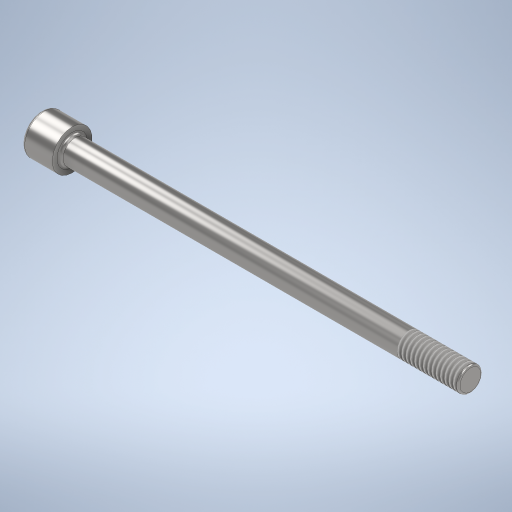
# Autodesk Inventor part: m4x70_example
Saved by Autodesk Inventor 2024 (Build 280153000, 153)
## iProperties
Created: 2025-12-19
Part Number: m4x70_example
Material: Stainless Steel
Document SubType Name: Modeling
Designer: schar
Density: 8 g/cm^3
Appearance: Semi-Polished
Author: schar
Autodesk Inventor part; units mm, degrees
ref_plane "YZ Plane" through (0, 0, 0) normal (1, 0, 0) x (0, 1, 0)
ref_plane "XZ Plane" through (0, 0, 0) normal (0, 1, 0) x (-1, 0, 0)
ref_plane "XY Plane" through (0, 0, 0) normal (0, 0, 1) x (1, 0, 0)
sketch "Sketch1" plane through (0, 0, 0) normal (1, 0, 0) x (0, 1, 0)
  circle A0 centre (0, 0) radius 3.25
  circle A1 centre (0, 0) radius 2
  dimension "d0" = 6.5
  dimension "d1" = 4
  constraints: 2 centre point, 2 coincident
  measures "d0" diameter of A0
  measures "d1" diameter of A1
extrude "Extrusion1" add sketch "Sketch1" along normal blind 5 contours A0 | A1
sketch "Sketch2" plane through (5, 0, 0) normal (1, 0, 0) x (0, 0, -1)
  circle A0 centre (0, 0) radius 2
  dimension "d4" = 4
  constraints: 1 centre point, 1 coincident
  measures "d4" diameter of A0
extrude "Extrusion2" add sketch "Sketch2" along normal blind 70
sketch "Sketch3" plane through (0, 0, 0) normal (-1, 0, 0) x (0, 0, 1)
  circle A0 centre (0, 0) radius 2 projected
  line L0 (2, -1.1547) -> (0, -2.3094)
  line L1 (0, -2.3094) -> (-2, -1.1547)
  line L2 (-2, -1.1547) -> (-2, 1.1547)
  line L3 (-2, 1.1547) -> (0, 2.3094)
  line L4 (0, 2.3094) -> (2, 1.1547)
  line L5 (2, 1.1547) -> (2, -1.1547)
  point P0 (2, 0)
  constraints: 12 end point, 1 coincident, 1 horizontal alignment, 1 midpoint, 14 other
extrude "Extrusion3" cut sketch "Sketch3" against normal blind 3.5
thread "Thread1" size "M4x0.7" class "6g" standard "ANSI Metric M Profile" length 15
fillet "Fillet1" radius 0.5 3 edges at (5, 0, 2) (0, -3.25, 0) (75, 0, 2)
sketch "Sketch4" plane through (75, 0, 0) normal (1, 0, 0) x (0, 0, -1)
  line L0 (-7.7054, 6.4284) -> (8.1646, 6.4284)
  line L1 (8.1646, 6.4284) -> (8.1646, -6.8875)
  line L2 (8.1646, -6.8875) -> (-7.7054, -6.8875)
  line L3 (-7.7054, -6.8875) -> (-7.7054, 6.4284)
  point P0 (0, 0)
  constraints: 8 end point, 2 parallel, 1 horizontal, 1 perpendicular
extrude "Extrusion4" cut sketch "Sketch4" against normal blind 5
fillet "Fillet2" radius 0.3 1 edges at (70, 0, 2)
body "Solid1"
